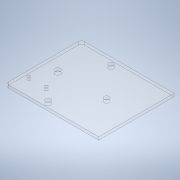
# Autodesk Inventor part: Tapa B1
Saved by Autodesk Inventor 2020.3 (Build 243373000, 373)
## iProperties
Created: 2020-07-27
Part Number: Tapa B1
Material: Polycarbonate, Clear
Document SubType Name: Modeling
Designer: juanp
Density: 1.2 g/cm^3
Appearance: Polycarbonate - Clear
Author: juanp
Autodesk Inventor part; units mm, degrees
ref_plane "YZ Plane" through (0, 0, 0) normal (1, 0, 0) x (0, 1, 0)
ref_plane "XZ Plane" through (0, 0, 0) normal (0, 1, 0) x (-1, 0, 0)
ref_plane "XY Plane" through (0, 0, 0) normal (0, 0, 1) x (1, 0, 0)
sketch "Sketch1" plane through (4, 0, 0) normal (0, 1, 0) x (-1, 0, 0)
  circle A0 centre (0, 0) radius 30.16 construction
  line L0 (0, 0) -> (38.16, 0) construction
  line L1 (38.16, 38.16) -> (38.16, -38.16) construction
  line L2 (38.16, 38.16) -> (-30.16, 38.16)
  line L3 (38.16, -38.16) -> (-30.16, -38.16)
  circle A1 centre (27.211, 31.78) radius 2.55
  circle A2 centre (27.211, -31.78) radius 2.55
  circle A3 centre (0, 0) radius 2.55
  line L4 (-30.16, 38.16) -> (-30.16, -38.16)
  line L5 (38.16, 0) -> (49.41, 0) construction
  circle A4 centre (49.41, 0) radius 2.75
  line L6 (40.66, 20.5) -> (58.16, 20.5) construction
  circle A5 centre (58.16, 20.5) radius 1.55
  circle A6 centre (40.66, 20.5) radius 1.55
  line L7 (49.41, 0) -> (63.66, 0) construction
  line L8 (38.16, -38.16) -> (63.66, -38.16)
  line L9 (63.66, -38.16) -> (63.66, 38.16)
  line L10 (63.66, 38.16) -> (38.16, 38.16)
  dimension "d6" = 60.32
  dimension "d4" = 38.16
  dimension "d5" = 76.32
  dimension "d1" = 5.1
  dimension "d3" = 6.38
  dimension "d2" = 10.949
  dimension "d0" = 5.1
  dimension "d10" = 11.25
  dimension "d11" = 5.5
  dimension "d12" = 17.66
  dimension "d13" = 2.5
  dimension "d14" = 17.5
  dimension "d15" = 3.1
  dimension "d16" = 3.1
  dimension "d17" = 14.25
  constraints: 22 end point, 7 centre point, 7 horizontal, 6 coincident, 2 midpoint, 2 perpendicular, 2 vertical, 1 symmetric about line, 1 tangent, 2 other
  measures "d6" diameter of A0
  measures "d4" distance of L0.end L0.start
  measures "d5" distance of L1.start L1.end
  measures "d1" diameter of A1
  measures "d3" distance from line of L2 A1.centre
  measures "d2" distance from line of L1 A1.centre
  measures "d0" diameter of A3
  measures "d10" distance of L0.end L5.end
  measures "d11" diameter of A4
  measures "d12" distance from line of L2 L6.start
  measures "d13" distance from line of L1 L6.start
  measures "d14" distance of L6.start L6.end
  measures "d15" diameter of A5
  measures "d16" diameter of A6
  measures "d17" distance of L7.start L7.end
extrude "Extrusion1" add sketch "Sketch1" along normal blind 3
fillet "Fillet1" radius 3 2 edges at (-59.66, 1.5, 38.16) (-59.66, 1.5, -38.16)
body "Solid1"
